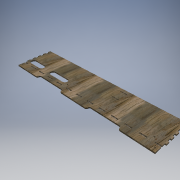
# Autodesk Inventor part: Dietro
Saved by Autodesk Inventor 2018.3 (Build 223284000, 284)
## iProperties
Created: 2019-03-05
Part Number: Dietro
Material: Generico
Document SubType Name: Modeling
Designer: AlfyPc
Density: 1 g/cm^3
Appearance: Legno alla deriva
Author: AlfyPc
Autodesk Inventor part; units mm, degrees
ref_plane "YZ Plane" through (0, 0, 0) normal (1, 0, 0) x (0, 1, 0)
ref_plane "XZ Plane" through (0, 0, 0) normal (0, 1, 0) x (-1, 0, 0)
ref_plane "XY Plane" through (0, 0, 0) normal (0, 0, 1) x (1, 0, 0)
sketch "Schizzo1" plane through (0, 0, 0) normal (0, 0, 1) x (1, 0, 0)
  line L0 (-15, -4) -> (-15, 0) construction
  line L1 (-34, 0) -> (-15, 0) construction
  line L2 (-53, 0) -> (-34, 0) construction
  line L3 (-72, 0) -> (-53, 0) construction
  line L4 (-91, 0) -> (-72, 0) construction
  line L5 (-110, 0) -> (-91, 0) construction
  line L6 (-129, 0) -> (-110, 0) construction
  line L7 (-148, 0) -> (-129, 0) construction
  line L8 (-167, 0) -> (-148, 0) construction
  line L9 (-186, 0) -> (-167, 0) construction
  line L10 (-205, 0) -> (-186, 0) construction
  line L11 (-224, 0) -> (-205, 0) construction
  line L12 (-243, 0) -> (-224, 0) construction
  line L13 (-262, 0) -> (-243, 0) construction
  line L14 (-281, 0) -> (-262, 0) construction
  line L15 (-300, 0) -> (-281, 0) construction
  line L16 (-319, 0) -> (-300, 0) construction
  line L17 (-338, 0) -> (-319, 0) construction
  line L18 (-357, 0) -> (-338, 0) construction
  line L19 (-376, 0) -> (-357, 0) construction
  line L20 (-395, 0) -> (-376, 0) construction
  line L21 (-414, 0) -> (-395, 0) construction
  line L22 (-433, 0) -> (-414, 0) construction
  line L23 (-452, 0) -> (-433, 0) construction
  line L24 (-471, 0) -> (-452, 0) construction
  line L25 (-471, -4) -> (-471, 0) construction
  line L26 (-452, -4) -> (-471, -4) construction
  line L27 (-452, 0) -> (-452, -4) construction
  line L28 (-15, -4) -> (-34, -4) construction
  line L29 (4, -4) -> (-15, -4) construction
  line L30 (4, 0) -> (4, -4) construction
  line L31 (-15, 0) -> (4, 0) construction
  line L32 (-34, 0) -> (-34, -4) construction
  line L33 (-53, -4) -> (-53, 0) construction
  line L34 (-34, -4) -> (-53, -4) construction
  line L35 (-72, 0) -> (-72, -4) construction
  line L36 (-53, -4) -> (-72, -4) construction
  line L37 (-91, -4) -> (-91, 0) construction
  line L38 (-72, -4) -> (-91, -4) construction
  line L39 (-110, 0) -> (-110, -4) construction
  line L40 (-91, -4) -> (-110, -4) construction
  line L41 (-129, -4) -> (-129, 0) construction
  line L42 (-110, -4) -> (-129, -4) construction
  line L43 (-148, 0) -> (-148, -4) construction
  line L44 (-129, -4) -> (-148, -4) construction
  line L45 (-167, -4) -> (-167, 0) construction
  line L46 (-148, -4) -> (-167, -4) construction
  line L47 (-186, 0) -> (-186, -4) construction
  line L48 (-167, -4) -> (-186, -4) construction
  line L49 (-205, -4) -> (-205, 0) construction
  line L50 (-186, -4) -> (-205, -4) construction
  line L51 (-224, 0) -> (-224, -4) construction
  line L52 (-205, -4) -> (-224, -4) construction
  line L53 (-243, -4) -> (-243, 0) construction
  line L54 (-224, -4) -> (-243, -4) construction
  line L55 (-262, 0) -> (-262, -4) construction
  line L56 (-243, -4) -> (-262, -4) construction
  line L57 (-281, -4) -> (-281, 0) construction
  line L58 (-262, -4) -> (-281, -4) construction
  line L59 (-300, 0) -> (-300, -4) construction
  line L60 (-281, -4) -> (-300, -4) construction
  line L61 (-319, -4) -> (-319, 0) construction
  line L62 (-300, -4) -> (-319, -4) construction
  line L63 (-338, 0) -> (-338, -4) construction
  line L64 (-319, -4) -> (-338, -4) construction
  line L65 (-357, -4) -> (-357, 0) construction
  line L66 (-338, -4) -> (-357, -4) construction
  line L67 (-376, 0) -> (-376, -4) construction
  line L68 (-357, -4) -> (-376, -4) construction
  line L69 (-395, -4) -> (-395, 0) construction
  line L70 (-376, -4) -> (-395, -4) construction
  line L71 (-414, 0) -> (-414, -4) construction
  line L72 (-395, -4) -> (-414, -4) construction
  line L73 (-433, -4) -> (-433, 0) construction
  line L74 (-414, -4) -> (-433, -4) construction
  line L75 (-433, -4) -> (-452, -4) construction
  line L76 (4, 95) -> (4, 0) construction
  line L77 (4, 0) -> (0, 0) construction
  line L78 (0, 0) -> (0, 95) construction
  line L79 (0, 95) -> (4, 95) construction
  line L80 (4, -4) -> (4, -24) construction
  line L81 (4, -24) -> (0, -24) construction
  line L82 (0, -24) -> (0, -4) construction
  line L83 (0, -4) -> (4, -4) construction
  line L84 (-381, -24) -> (-471, -24)
  line L85 (-471, -24) -> (-471, 95)
  line L86 (-471, 95) -> (4, 95)
  line L87 (4, 95) -> (4, -24)
  line L88 (-376, -19) -> (-376, -19)
  line L89 (-371, -14) -> (-286, -14)
  line L90 (-281, -19) -> (-281, -19)
  line L91 (-276, -24) -> (-191, -24)
  arc A0 (-381, -24) -> (-376, -19) centre (-381, -19) ccw
  arc A1 (-371, -14) -> (-376, -19) centre (-371, -19) ccw
  arc A2 (-281, -19) -> (-286, -14) centre (-286, -19) ccw
  arc A3 (-281, -19) -> (-276, -24) centre (-276, -19) ccw
  line L92 (-186, -19) -> (-186, -19)
  line L93 (-181, -14) -> (-96, -14)
  line L94 (-91, -19) -> (-91, -19)
  line L95 (-86, -24) -> (4, -24)
  arc A4 (-191, -24) -> (-186, -19) centre (-191, -19) ccw
  arc A5 (-181, -14) -> (-186, -19) centre (-181, -19) ccw
  arc A6 (-91, -19) -> (-96, -14) centre (-96, -19) ccw
  arc A7 (-91, -19) -> (-86, -24) centre (-86, -19) ccw
  line L96 (-15, -4) -> (4, -4) projected
  line L97 (4, 0) -> (4, -4) projected
  line L98 (4, 0) -> (-15, 0) projected
  line L99 (-15, 0) -> (-15, -4) projected
  line L100 (-53, -4) -> (-34, -4) projected
  line L101 (-34, 0) -> (-34, -4) projected
  line L102 (-53, 0) -> (-34, 0) projected
  line L103 (-53, 0) -> (-53, -4) projected
  line L104 (-91, -4) -> (-72, -4) projected
  line L105 (-72, 0) -> (-72, -4) projected
  line L106 (-91, 0) -> (-72, 0) projected
  line L107 (-91, 0) -> (-91, -4) projected
  line L108 (-129, -4) -> (-110, -4) projected
  line L109 (-110, 0) -> (-110, -4) projected
  line L110 (-129, 0) -> (-110, 0) projected
  line L111 (-129, 0) -> (-129, -4) projected
  line L112 (-167, -4) -> (-148, -4) projected
  line L113 (-148, 0) -> (-148, -4) projected
  line L114 (-167, 0) -> (-148, 0) projected
  line L115 (-167, 0) -> (-167, -4) projected
  line L116 (-205, -4) -> (-186, -4) projected
  line L117 (-186, 0) -> (-186, -4) projected
  line L118 (-205, 0) -> (-186, 0) projected
  line L119 (-205, 0) -> (-205, -4) projected
  line L120 (-243, -4) -> (-224, -4) projected
  line L121 (-224, 0) -> (-224, -4) projected
  line L122 (-243, 0) -> (-224, 0) projected
  line L123 (-243, 0) -> (-243, -4) projected
  line L124 (-281, -4) -> (-262, -4) projected
  line L125 (-262, 0) -> (-262, -4) projected
  line L126 (-281, 0) -> (-262, 0) projected
  line L127 (-281, 0) -> (-281, -4) projected
  line L128 (-319, -4) -> (-300, -4) projected
  line L129 (-300, 0) -> (-300, -4) projected
  line L130 (-319, 0) -> (-300, 0) projected
  line L131 (-319, 0) -> (-319, -4) projected
  line L132 (-357, -4) -> (-338, -4) projected
  line L133 (-338, 0) -> (-338, -4) projected
  line L134 (-357, 0) -> (-338, 0) projected
  line L135 (-357, 0) -> (-357, -4) projected
  line L136 (-395, -4) -> (-376, -4) projected
  line L137 (-376, 0) -> (-376, -4) projected
  line L138 (-395, 0) -> (-376, 0) projected
  line L139 (-395, 0) -> (-395, -4) projected
  line L140 (-433, -4) -> (-414, -4) projected
  line L141 (-414, 0) -> (-414, -4) projected
  line L142 (-433, 0) -> (-414, 0) projected
  line L143 (-433, 0) -> (-433, -4) projected
  line L144 (-471, -4) -> (-452, -4) projected
  line L145 (-452, 0) -> (-452, -4) projected
  line L146 (-471, 0) -> (-452, 0) projected
  line L147 (-471, 0) -> (-471, -4) projected
  line L148 (-361.5, 18) -> (-309.6633, 18) construction
  line L149 (-361.5, 8.6924) -> (-309.6633, 8.6924)
  line L150 (-309.6633, 27.3076) -> (-361.5, 27.3076)
  arc A8 (-361.5, 27.3076) -> (-361.5, 8.6924) centre (-361.5, 18) ccw
  arc A9 (-309.6633, 8.6924) -> (-309.6633, 27.3076) centre (-309.6633, 18) ccw
  line L151 (-451.5, 18) -> (-411.5, 18) construction
  line L152 (-451.5, 28) -> (-411.5, 28)
  line L153 (-411.5, 8) -> (-451.5, 8)
  arc A10 (-451.5, 28) -> (-451.5, 8) centre (-451.5, 18) ccw
  arc A11 (-411.5, 8) -> (-411.5, 28) centre (-411.5, 18) ccw
  point P0 (-376, -14)
  point P1 (-281, -14)
  point P2 (-281, -24)
  point P3 (-186, -24)
  point P4 (-186, -14)
  point P5 (-91, -14)
  point P6 (-335.5816, 18)
  point P7 (-431.5, 18)
  dimension "d2" = 95
  dimension "d3" = 90
  dimension "d4" = 95
  dimension "d5" = 5
  dimension "d6" = 90
  dimension "d7" = 95
  dimension "d8" = 5
  dimension "d22" = 40
  dimension "d23" = 18
  dimension "d24" = 20
  dimension "d25" = 50
  constraints: 208 end point, 56 horizontal, 31 vertical, 24 point on circle, 24 tangent, 17 point on line, 12 centre point, 6 equal radius, 6 perpendicular, 4 parallel, 2 midpoint, 57 other
  measures "d2" distance of point (-376, -14) point (-281, -14)
  measures "d3" angle of L88 L89
  measures "d4" distance of point (-281, -24) point (-186, -24)
  measures "d5" radius of A0
  measures "d6" distance of L84.start L84.end
  measures "d7" distance of point (-186, -14) point (-91, -14)
  measures "d8" radius of A4
  measures "d22" distance of L151.start L151.end
  measures "d23" distance between parallel lines of L22 L151
  measures "d24" distance between parallel lines of L153 L152
  measures "d25" distance of L151.end L148.start
extrude "Estrusione1" add sketch "Schizzo1" along normal blind 4 contours L84 L85 L144 L145 L146 L86 L87 L98 L99 L96 L95 A7 A6 L93 A5 A4 L91 A3 A2 L89 A1 A0
sketch "Schizzo2" plane through (0, 0, 4) normal (0, 0, 1) x (1, 0, 0)
  line L0 (0, -4) -> (0, -24) projected
  line L1 (0, -24) -> (4, -24) projected
  line L2 (4, -4) -> (4, -24) projected
  line L3 (0, -4) -> (4, -4) projected
  line L4 (0, -4) -> (0, -24) construction
  line L5 (4, -4) -> (4, -24) construction
  line L6 (-467, -4) -> (-471, -4) projected
  line L7 (-471, -24) -> (-471, -4) projected
  line L8 (-467, -24) -> (-471, -24) projected
  line L9 (-467, -24) -> (-467, -4) projected
  line L10 (-467, 0) -> (-467, 9.5) construction
  line L11 (-471, 0) -> (-471, 9.5) construction
  line L12 (4, 0) -> (4, 95) projected
  line L13 (0, 0) -> (4, 0)
  line L14 (4, 0) -> (4, 9.5)
  line L15 (4, 9.5) -> (0, 9.5)
  line L16 (0, 9.5) -> (0, 0)
  line L17 (-471, 95) -> (-471, 0) projected
  line L18 (-467, 0) -> (-471, 0)
  line L19 (-471, 0) -> (-471, 9.5)
  line L20 (-471, 9.5) -> (-467, 9.5)
  line L21 (-467, 9.5) -> (-467, 0)
  line L22 (0, 19) -> (0, 9.5)
  line L23 (0, 9.5) -> (4, 9.5)
  line L24 (4, 9.5) -> (4, 19)
  line L25 (4, 19) -> (0, 19)
  line L26 (-467, 19) -> (-467, 9.5)
  line L27 (-467, 9.5) -> (-471, 9.5)
  line L28 (-471, 9.5) -> (-471, 19)
  line L29 (-471, 19) -> (-467, 19)
  line L30 (0, 28.5) -> (0, 19)
  line L31 (0, 19) -> (4, 19)
  line L32 (4, 19) -> (4, 28.5)
  line L33 (4, 28.5) -> (0, 28.5)
  line L34 (-467, 28.5) -> (-467, 19)
  line L35 (-467, 19) -> (-471, 19)
  line L36 (-471, 19) -> (-471, 28.5)
  line L37 (-471, 28.5) -> (-467, 28.5)
  line L38 (0, 38) -> (0, 28.5)
  line L39 (0, 28.5) -> (4, 28.5)
  line L40 (4, 28.5) -> (4, 38)
  line L41 (4, 38) -> (0, 38)
  line L42 (-467, 38) -> (-467, 28.5)
  line L43 (-467, 28.5) -> (-471, 28.5)
  line L44 (-471, 28.5) -> (-471, 38)
  line L45 (-471, 38) -> (-467, 38)
  line L46 (0, 47.5) -> (0, 38)
  line L47 (0, 38) -> (4, 38)
  line L48 (4, 38) -> (4, 47.5)
  line L49 (4, 47.5) -> (0, 47.5)
  line L50 (-467, 47.5) -> (-467, 38)
  line L51 (-467, 38) -> (-471, 38)
  line L52 (-471, 38) -> (-471, 47.5)
  line L53 (-471, 47.5) -> (-467, 47.5)
  line L54 (0, 57) -> (0, 47.5)
  line L55 (0, 47.5) -> (4, 47.5)
  line L56 (4, 47.5) -> (4, 57)
  line L57 (4, 57) -> (0, 57)
  line L58 (-467, 57) -> (-467, 47.5)
  line L59 (-467, 47.5) -> (-471, 47.5)
  line L60 (-471, 47.5) -> (-471, 57)
  line L61 (-471, 57) -> (-467, 57)
  line L62 (0, 66.5) -> (0, 57)
  line L63 (0, 57) -> (4, 57)
  line L64 (4, 57) -> (4, 66.5)
  line L65 (4, 66.5) -> (0, 66.5)
  line L66 (-467, 66.5) -> (-467, 57)
  line L67 (-467, 57) -> (-471, 57)
  line L68 (-471, 57) -> (-471, 66.5)
  line L69 (-471, 66.5) -> (-467, 66.5)
  line L70 (0, 76) -> (0, 66.5)
  line L71 (0, 66.5) -> (4, 66.5)
  line L72 (4, 66.5) -> (4, 76)
  line L73 (4, 76) -> (0, 76)
  line L74 (-467, 76) -> (-467, 66.5)
  line L75 (-467, 66.5) -> (-471, 66.5)
  line L76 (-471, 66.5) -> (-471, 76)
  line L77 (-471, 76) -> (-467, 76)
  line L78 (0, 85.5) -> (0, 76)
  line L79 (0, 76) -> (4, 76)
  line L80 (4, 76) -> (4, 85.5)
  line L81 (4, 85.5) -> (0, 85.5)
  line L82 (-467, 85.5) -> (-467, 76)
  line L83 (-467, 76) -> (-471, 76)
  line L84 (-471, 76) -> (-471, 85.5)
  line L85 (-471, 85.5) -> (-467, 85.5)
  line L86 (0, 95) -> (0, 85.5)
  line L87 (0, 85.5) -> (4, 85.5)
  line L88 (4, 85.5) -> (4, 95)
  line L89 (4, 95) -> (0, 95)
  line L90 (-467, 95) -> (-467, 85.5)
  line L91 (-467, 85.5) -> (-471, 85.5)
  line L92 (-471, 85.5) -> (-471, 95)
  line L93 (-471, 95) -> (-467, 95)
  line L94 (0, -24) -> (4, -24) projected
  line L95 (0, -4) -> (4, -4) projected
  line L96 (-467, 9.5) -> (-471, 9.5) projected
  line L97 (-471, 0) -> (-467, 0) projected
  point P0 (4, 9.5)
  point P1 (-471, 9.5)
  point P2 (4, 19)
  point P3 (-471, 19)
  point P4 (4, 28.5)
  point P5 (-471, 28.5)
  point P6 (4, 38)
  point P7 (-471, 38)
  point P8 (4, 47.5)
  point P9 (-471, 47.5)
  point P10 (4, 57)
  point P11 (-471, 57)
  point P12 (4, 66.5)
  point P13 (-471, 66.5)
  point P14 (4, 76)
  point P15 (-471, 76)
  point P16 (4, 85.5)
  point P17 (-471, 85.5)
  point P18 (-471, 9.5)
  dimension "d11" = 9.5
  dimension "d12" = 9.5
  dimension "d15" = 9.5
  constraints: 160 end point, 4 parallel, 2 horizontal, 2 perpendicular, 2 point on line, 1 vertical, 162 other
  measures "d11" distance of L14.end L13.end
  measures "d12" distance of L18.end L11.end
  measures "d15" distance of L13.start L22.end
extrude "Estrusione2" cut sketch "Schizzo2" against normal blind 4 contours L3 L2 L1 L0 | L9 L8 L7 L6 | L13 L16 L15 L12 | L25 L30 L33 L12 | L41 L46 L49 L12 | L57 L62 L65 L12 | L73 L78 L81 L12 | L85 L82 L77 L17 | L69 L66 L61 L17 | L53 L50 L45 L17 | L37 L34 L29 L17 | L20 L21 L18 L17
sketch "Schizzo3" plane through (0, 0, 4) normal (0, 0, 1) x (1, 0, 0)
  line L0 (-444.15, 0) -> (-440.85, 0) projected
  line L1 (-292.15, 0) -> (-288.85, 0) projected
  line L2 (-26.15, 0) -> (-22.85, 0) projected
  line L3 (-442.5, 0) -> (-442.5, 5) construction
  line L4 (-442.5, 0) -> (-437.5, 0) construction
  line L5 (-290.5, 0) -> (-290.5, 10) construction
  circle A0 centre (-442.5, 5) radius 1.65
  circle A1 centre (-290.5, 10) radius 1.65
  line L6 (-24.5, 0) -> (-24.5, 10) construction
  circle A2 centre (-24.5, 10) radius 1.65
  line L7 (0, -24) -> (0, -4) projected
  line L8 (0, -4) -> (-15, -4) projected
  line L9 (-15, -4) -> (-15, 0) projected
  line L10 (-15, 0) -> (0, 0) projected
  line L11 (0, 0) -> (0, 9.5) projected
  line L12 (0, 9.5) -> (4, 9.5) projected
  line L13 (4, 9.5) -> (4, 19) projected
  line L14 (4, 19) -> (0, 19) projected
  line L15 (0, 19) -> (0, 28.5) projected
  line L16 (0, 28.5) -> (4, 28.5) projected
  line L17 (4, 28.5) -> (4, 38) projected
  line L18 (4, 38) -> (0, 38) projected
  line L19 (0, 38) -> (0, 47.5) projected
  line L20 (0, 47.5) -> (4, 47.5) projected
  line L21 (4, 47.5) -> (4, 57) projected
  line L22 (4, 57) -> (0, 57) projected
  line L23 (0, 57) -> (0, 66.5) projected
  line L24 (0, 66.5) -> (4, 66.5) projected
  line L25 (4, 66.5) -> (4, 76) projected
  line L26 (4, 76) -> (0, 76) projected
  line L27 (0, 76) -> (0, 85.5) projected
  line L28 (0, 85.5) -> (4, 85.5) projected
  line L29 (4, 85.5) -> (4, 95) projected
  line L30 (4, 95) -> (-471, 95) projected
  line L31 (-471, 95) -> (-471, 85.5) projected
  line L32 (-471, 85.5) -> (-467, 85.5) projected
  line L33 (-467, 85.5) -> (-467, 76) projected
  line L34 (-467, 76) -> (-471, 76) projected
  line L35 (-471, 76) -> (-471, 66.5) projected
  line L36 (-471, 66.5) -> (-467, 66.5) projected
  line L37 (-467, 66.5) -> (-467, 57) projected
  line L38 (-467, 57) -> (-471, 57) projected
  line L39 (-471, 57) -> (-471, 47.5) projected
  line L40 (-471, 47.5) -> (-467, 47.5) projected
  line L41 (-467, 47.5) -> (-467, 38) projected
  line L42 (-467, 38) -> (-471, 38) projected
  line L43 (-471, 38) -> (-471, 28.5) projected
  line L44 (-471, 28.5) -> (-467, 28.5) projected
  line L45 (-467, 28.5) -> (-467, 19) projected
  line L46 (-467, 19) -> (-471, 19) projected
  line L47 (-471, 19) -> (-471, 9.5) projected
  line L48 (-471, 9.5) -> (-467, 9.5) projected
  line L49 (-467, 9.5) -> (-467, 0) projected
  line L50 (-467, 0) -> (-452, 0) projected
  line L51 (-452, 0) -> (-452, -4) projected
  line L52 (-452, -4) -> (-467, -4) projected
  line L53 (-467, -4) -> (-467, -24) projected
  line L54 (-467, -24) -> (-381, -24) projected
  arc A3 (-381, -24) -> (-376, -19) centre (-381, -19) ccw projected
  arc A4 (-371, -14) -> (-376, -19) centre (-371, -19) ccw projected
  line L55 (-371, -14) -> (-286, -14) projected
  arc A5 (-281, -19) -> (-286, -14) centre (-286, -19) ccw projected
  arc A6 (-281, -19) -> (-276, -24) centre (-276, -19) ccw projected
  line L56 (-276, -24) -> (-191, -24) projected
  arc A7 (-191, -24) -> (-186, -19) centre (-191, -19) ccw projected
  arc A8 (-181, -14) -> (-186, -19) centre (-181, -19) ccw projected
  line L57 (-181, -14) -> (-96, -14) projected
  arc A9 (-91, -19) -> (-96, -14) centre (-96, -19) ccw projected
  arc A10 (-91, -19) -> (-86, -24) centre (-86, -19) ccw projected
  line L58 (-86, -24) -> (0, -24) projected
  arc A11 (-361.5, 27.3076) -> (-361.5, 8.6924) centre (-361.5, 18) ccw projected
  line L59 (-361.5, 27.3076) -> (-309.6633, 27.3076) projected
  arc A12 (-309.6633, 8.6924) -> (-309.6633, 27.3076) centre (-309.6633, 18) ccw projected
  line L60 (-309.6633, 8.6924) -> (-361.5, 8.6924) projected
  arc A13 (-411.5, 8) -> (-411.5, 28) centre (-411.5, 18) ccw projected
  line L61 (-411.5, 8) -> (-451.5, 8) projected
  arc A14 (-451.5, 28) -> (-451.5, 8) centre (-451.5, 18) ccw projected
  line L62 (-451.5, 28) -> (-411.5, 28) projected
  line L63 (-34, -4) -> (-53, -4) projected
  line L64 (-53, -4) -> (-53, 0) projected
  line L65 (-53, 0) -> (-34, 0) projected
  line L66 (-34, 0) -> (-34, -4) projected
  line L67 (-72, -4) -> (-91, -4) projected
  line L68 (-91, -4) -> (-91, 0) projected
  line L69 (-91, 0) -> (-72, 0) projected
  line L70 (-72, 0) -> (-72, -4) projected
  line L71 (-110, -4) -> (-129, -4) projected
  line L72 (-129, -4) -> (-129, 0) projected
  line L73 (-129, 0) -> (-110, 0) projected
  line L74 (-110, 0) -> (-110, -4) projected
  line L75 (-148, -4) -> (-167, -4) projected
  line L76 (-167, -4) -> (-167, 0) projected
  line L77 (-167, 0) -> (-148, 0) projected
  line L78 (-148, 0) -> (-148, -4) projected
  line L79 (-186, -4) -> (-205, -4) projected
  line L80 (-205, -4) -> (-205, 0) projected
  line L81 (-205, 0) -> (-186, 0) projected
  line L82 (-186, 0) -> (-186, -4) projected
  line L83 (-224, -4) -> (-243, -4) projected
  line L84 (-243, -4) -> (-243, 0) projected
  line L85 (-243, 0) -> (-224, 0) projected
  line L86 (-224, 0) -> (-224, -4) projected
  line L87 (-262, -4) -> (-281, -4) projected
  line L88 (-281, -4) -> (-281, 0) projected
  line L89 (-281, 0) -> (-262, 0) projected
  line L90 (-262, 0) -> (-262, -4) projected
  line L91 (-300, -4) -> (-319, -4) projected
  line L92 (-319, -4) -> (-319, 0) projected
  line L93 (-319, 0) -> (-300, 0) projected
  line L94 (-300, 0) -> (-300, -4) projected
  line L95 (-338, -4) -> (-357, -4) projected
  line L96 (-357, -4) -> (-357, 0) projected
  line L97 (-357, 0) -> (-338, 0) projected
  line L98 (-338, 0) -> (-338, -4) projected
  line L99 (-376, -4) -> (-395, -4) projected
  line L100 (-395, -4) -> (-395, 0) projected
  line L101 (-395, 0) -> (-376, 0) projected
  line L102 (-376, 0) -> (-376, -4) projected
  line L103 (-414, -4) -> (-433, -4) projected
  line L104 (-433, -4) -> (-433, 0) projected
  line L105 (-433, 0) -> (-414, 0) projected
  line L106 (-414, 0) -> (-414, -4) projected
  line L107 (-467, 85.5) -> (-467, 76) construction
  line L108 (-467, 80.75) -> (-460, 80.75) construction
  line L109 (0, 85.5) -> (0, 76) construction
  line L110 (0, 80.75) -> (-7, 80.75) construction
  line L111 (0, -4) -> (0, -24) construction
  line L112 (0, -14) -> (-7, -14) construction
  line L113 (-467, -24) -> (-467, -4) construction
  line L114 (-467, -14) -> (-460, -14) construction
  circle A15 centre (-460, -14) radius 1.65
  circle A16 centre (-460, 80.75) radius 1.65
  circle A17 centre (-7, 80.75) radius 1.65
  circle A18 centre (-7, -14) radius 1.65
  dimension "d26" = 5
  dimension "d27" = 90
  dimension "d28" = 10
  dimension "d29" = 3.3
  dimension "d30" = 3.3
  dimension "d31" = 10
  dimension "d32" = 3.3
  dimension "d38" = 7
  dimension "d39" = 7
  dimension "d40" = 7
  dimension "d41" = 7
  dimension "d42" = 3.3
  dimension "d43" = 3.3
  dimension "d44" = 3.3
  dimension "d45" = 3.3
  constraints: 16 end point, 7 centre point, 7 coincident, 7 midpoint, 5 horizontal, 3 vertical, 1 perpendicular
  measures "d26" distance of L3.start L3.end
  measures "d27" angle of L4 L3
  measures "d28" distance of L5.start L5.end
  measures "d29" diameter of A0
  measures "d30" diameter of A1
  measures "d31" distance of L6.start L6.end
  measures "d32" diameter of A2
  measures "d38" distance of L108.start L108.end
  measures "d39" distance of L110.start L110.end
  measures "d40" distance of L112.start L112.end
  measures "d41" distance of L114.start L114.end
  measures "d42" diameter of A15
  measures "d43" diameter of A16
  measures "d44" diameter of A17
  measures "d45" diameter of A18
extrude "Estrusione3" cut sketch "Schizzo3" against normal blind 4 contours A0 | A1 | A2 | A15 | A16 | A17 | A18
sketch "Schizzo5" plane through (0, 0, 0) normal (0, 0, -1) x (-1, 0, 0)
  line L0 (154, 85) -> (174, 85)
  line L1 (174, 85) -> (174, 82)
  line L2 (174, 82) -> (154, 82)
  line L3 (154, 82) -> (154, 85)
  line L4 (174, 51) -> (154, 51)
  line L5 (154, 51) -> (154, 54)
  line L6 (154, 54) -> (174, 54)
  line L7 (174, 54) -> (174, 51)
  point P0 (0, 0)
  dimension "d35" = 3
  constraints: 16 end point, 4 parallel, 2 horizontal, 2 perpendicular
  measures "d35" distance of L4.end L5.end
extrude "Estrusione4" cut sketch "Schizzo5" against normal blind 11.25
